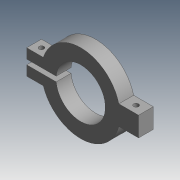
# Autodesk Inventor part: mallet_holder
Saved by Autodesk Inventor 2015 (Build 190159000, 159)
## iProperties
Created: 2014-08-31
Part Number: mallet_holder
Material: Generic
Document SubType Name: Modeling
Designer: shohei
Density: 1 g/cm^3
Appearance: Default
Author: shohei
Autodesk Inventor part; units mm, degrees
ref_plane "YZ Plane" through (0, 0, 0) normal (1, 0, 0) x (0, 1, 0)
ref_plane "XZ Plane" through (0, 0, 0) normal (0, 1, 0) x (-1, 0, 0)
ref_plane "XY Plane" through (0, 0, 0) normal (0, 0, 1) x (1, 0, 0)
sketch "Sketch1" plane through (0, 0, 0) normal (0, 1, 0) x (-1, 0, 0)
  arc A0 (49.7494, 5) -> (49.7494, -5) centre (0, 0) ccw
  line L0 (49.7494, 5) -> (109.7494, 5)
  line L1 (109.7494, 5) -> (109.7494, 25)
  line L2 (155.1912, 0) -> (-162.9015, 0) projected
  line L3 (0, -115.4406) -> (0, 115.4406) projected
  line L4 (109.7494, 25) -> (75.9934, 25)
  line L5 (49.7494, -5) -> (109.7494, -5)
  line L6 (109.7494, -5) -> (109.7494, -25)
  line L7 (109.7494, -25) -> (75.9934, -25)
  line L8 (-77.4597, 20) -> (-117.4597, 20)
  line L9 (-117.4597, 20) -> (-117.4597, 0)
  line L10 (-77.4597, -20) -> (-117.4597, -20)
  line L11 (-117.4597, -20) -> (-117.4597, 0)
  arc A1 (75.9934, 25) -> (-77.4597, 20) centre (0, 0) ccw
  arc A2 (-77.4597, -20) -> (75.9934, -25) centre (0, 0) ccw
  point P0 (43.3013, 25)
  point P1 (43.3013, -25)
  dimension "d0" = 100
  dimension "d4" = 5
  dimension "d5" = 20
  dimension "d13" = 20
  dimension "d14" = 40
  dimension "d20" = 60
  constraints: 20 end point, 7 point on circle, 6 symmetric about line, 3 centre point, 3 horizontal, 2 coincident, 1 perpendicular, 1 point on line, 1 vertical
  measures "d0" diameter of A0
  measures "d4" distance between parallel lines of L2 L0
  measures "d5" distance of L0.end L1.end
  measures "d13" distance between parallel lines of L2 L8
  measures "d14" distance of L8.start L8.end
  measures "d20" distance of L5.start L6.start
extrude "Extrusion1" add sketch "Sketch1" along normal blind 30 contours A0 L3 A1 L4 L1 L0 | A0 L2 L9 L8 A1 L3 | A0 L3 A2 L10 L11 L2 | A0 L5 L6 L7 A2 L3
sketch "Sketch3" plane through (-109.7494, 0, 25) normal (0, 0, 1) x (1, 0, 0)
  circle A0 centre (15, 15) radius 5
  line L0 (0, 0) -> (33.756, 0) projected
  line L1 (0, 0) -> (0, 30) projected
  point P0 (109.7494, 0)
  dimension "d8" = 10
  dimension "d9" = 15
  dimension "d10" = 15
  constraints: 1 centre point
  measures "d8" diameter of A0
  measures "d9" distance from line of L0 A0.centre
  measures "d10" distance from line of L1 A0.centre
extrude "Extrusion2" cut sketch "Sketch3" against normal through all
sketch "Sketch4" plane through (117.4597, 0, -20) normal (0, 0, -1) x (-1, 0, 0)
  circle A0 centre (20, 15) radius 5
  line L0 (0, 0) -> (0, 30) projected
  line L1 (0, 30) -> (40, 30) projected
  point P0 (117.4597, 0)
  dimension "d15" = 10
  dimension "d16" = 20
  dimension "d17" = 15
  constraints: 1 centre point
  measures "d15" diameter of A0
  measures "d16" distance from line of L0 A0.centre
  measures "d17" distance from line of L1 A0.centre
extrude "Extrusion3" cut sketch "Sketch4" against normal through all
equation "\"d0\" = Grip"
equation "\"Grip\" = 100"
body "Solid1"
